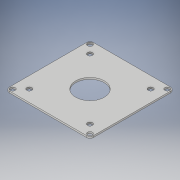
# Autodesk Inventor part: POWER_distribution
Saved by Autodesk Inventor 2019 (Build 230136000, 136)
## iProperties
Created: 2020-03-13
Part Number: POWER_distribution
Material: Generic
Document SubType Name: Modeling
Designer: Pulag
Density: 1 g/cm^3
Appearance: Default
Author: Pulag
Autodesk Inventor part; units mm, degrees
ref_plane "YZ Plane" through (0, 0, 0) normal (1, 0, 0) x (0, 1, 0)
ref_plane "XZ Plane" through (0, 0, 0) normal (0, 1, 0) x (-1, 0, 0)
ref_plane "XY Plane" through (0, 0, 0) normal (0, 0, 1) x (1, 0, 0)
sketch "Sketch1" plane through (0, 0, 0) normal (0, 1, 0) x (-1, 0, 0)
  line L0 (0, 25) -> (25, 25)
  line L1 (25, 25) -> (25, 0)
  line L2 (25, 25) -> (23, 25)
  line L3 (25, 23) -> (25, 25)
  circle A0 centre (23, 23) radius 1.5
  circle A1 centre (18.0503, 18.0503) radius 1.5
  line L4 (0, 25) -> (0, 8.5)
  line L5 (8.5, 0) -> (25, 0)
  arc A2 (8.5, 0) -> (0, 8.5) centre (0, 0) ccw
  dimension "d5" = 3
  dimension "d7" = 3
  constraints: 12 end point, 3 centre point, 2 coincident, 2 horizontal, 2 point on circle, 1 perpendicular, 1 vertical
  measures "d5" diameter of A0
  measures "d7" diameter of A1
extrude "Extrusion1" add sketch "Sketch1" along normal blind 1
pattern_circular "Circular Pattern1" count 4 over 360 about axis through (0, 0, 0) along (0, 1, 0) of "Extrusion1"
fillet "Fillet1" radius 2 4 edges at (-25, 0.5, 25) (-25, 0.5, -25) (25, 0.5, 25) (25, 0.5, -25)
body "Solid1"
